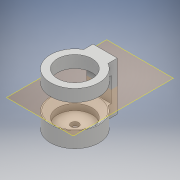
# Autodesk Inventor part: baseRotor1
Saved by Autodesk Inventor 2017 (Build 210142000, 142)
## iProperties
Created: 2017-08-06
Part Number: baseRotor1
Material: Generic
Document SubType Name: Sheet Metal
Designer: Bardo91
Density: 1 g/cm^3
Sheet Metal Rule: Default_mm
Appearance: Default
Author: Bardo91
Autodesk Inventor part; units mm, degrees
ref_plane "YZ Plane" through (0, 0, 0) normal (1, 0, 0) x (0, 1, 0)
ref_plane "XZ Plane" through (0, 0, 0) normal (0, 1, 0) x (-1, 0, 0)
ref_plane "XY Plane" through (0, 0, 0) normal (0, 0, 1) x (1, 0, 0)
sketch "Sketch1" plane through (0, 0, 0) normal (0, 0, 1) x (1, 0, 0)
  circle A0 centre (0, 0) radius 14.25
  circle A1 centre (0, 0) radius 20
  line L0 (0, 20) -> (10, 20)
  line L1 (10, 20) -> (10, 17.3205)
  line L2 (0, 20) -> (0, 20)
  line L3 (0, 20) -> (-10, 20)
  line L4 (-10, 20) -> (-10, 17.3205)
  point P0 (-20, 0)
  point P1 (20, 0)
  dimension "d0" = 28.5
  dimension "d1" = 40
  dimension "d25" = 10
  dimension "d31" = 10
  dimension "d32" = 0
  constraints: 10 end point, 5 point on circle, 2 centre point, 2 coincident, 2 perpendicular, 1 horizontal
  measures "d0" diameter of A0
  measures "d1" diameter of A1
  measures "d25" distance of L0.end L0.start
  measures "d31" distance of L0.start L3.end
  measures "d32" distance of L2.start L0.start
extrude "Extrusion1" add sketch "Sketch1" along normal blind 10
ref_plane "Work Plane1" through (0, 0, -10) normal (0, 0, 1) x (1, 0, 0)
mirror "Mirror1" about plane through (0, 0, -10) normal (0, 0, 1) of "Extrusion1"
sketch "Sketch2" plane through (0, 0, -30) normal (0, 0, -1) x (-1, 0, 0)
  circle A0 centre (0, 0) radius 14.25 projected
  circle A1 centre (0, 0) radius 20
  dimension "d11" = 40
  constraints: 1 centre point, 1 coincident
  measures "d11" diameter of A1
extrude "Extrusion2" add sketch "Sketch2" along normal blind 3 contours A0 | A1
sketch "Sketch3" plane through (0, 0, -30) normal (0, 0, 1) x (1, 0, 0)
  circle A0 centre (0, 0) radius 3.15
  dimension "d14" = 6.3
  constraints: 1 centre point, 1 coincident
  measures "d14" diameter of A0
extrude "Extrusion3" cut sketch "Sketch3" against normal blind 1
sketch "Sketch4" plane through (0, 0, -31) normal (0, 0, 1) x (1, 0, 0)
  circle A0 centre (0, 0) radius 3.15
  line L0 (0, 0) -> (0, -1.6)
  line L1 (0, -1.6) -> (-2.7134, -1.6)
  line L2 (0, -1.6) -> (2.7134, -1.6)
  dimension "d17" = 6.3
  dimension "d18" = 1.6
  constraints: 6 end point, 2 horizontal, 2 point on circle, 1 centre point, 1 coincident, 1 vertical
  measures "d17" diameter of A0
  measures "d18" distance of L0.start L0.end
extrude "Extrusion4" cut sketch "Sketch4" against normal through all contours A0 L2 L1 picked at (-0.0447, 1.5505)
sketch "Sketch6" plane through (-7.5, 20, -22) normal (0, 1, 0) x (1, 0, 0)
  line L0 (17.5, 8) -> (17.5, 8) projected
  line L1 (17.5, -22) -> (17.5, -32) projected
  line L2 (-2.5, 8) -> (17.5, 8)
  line L3 (17.5, 8) -> (17.5, -32)
  line L4 (17.5, -32) -> (-2.5, -32)
  line L5 (-2.5, -32) -> (-2.5, 8)
  point P0 (7.5, -22)
  constraints: 8 end point, 2 parallel, 1 horizontal, 1 horizontal alignment, 1 perpendicular
extrude "Extrusion6" add sketch "Sketch6" along normal blind 5
sketch "Sketch7" plane through (-7.5, 25, -22) normal (0, 1, 0) x (1, 0, 0)
  line L0 (21.75, -32) -> (-6.75, -32) projected
  line L1 (7.5, -32) -> (7.5, 8)
  line L2 (10.65, 8) -> (4.35, 8) projected
  circle A0 centre (7.5, -12) radius 4.25
  point P0 (7.5, -22)
  dimension "d28" = 8.5
  constraints: 3 midpoint, 2 end point, 1 centre point
  measures "d28" diameter of A0
extrude "Extrusion7" cut sketch "Sketch7" against normal up to next
chamfer "Chamfer1" distance 5 angle 45 1 edges at (-14.25, 0, -20)
equation "\"d4\" = d25"
equation "\"BendRadius\" = Thickness"
equation "\"BendReliefWidth\" = Thickness"
equation "\"BendReliefDepth\" = 0.5 * Thickness"
equation "\"CornerReliefSize\" = 4 * Thickness"
equation "\"MinimumRemnant\" = 2 * Thickness"
equation "\"TransitionRadius\" = BendRadius"
equation "\"JacobiRadiusSize\" = BendRadius"
equation "\"GapSize\" = Thickness"
equation "\"Thickness\" = 0.5"
body "Solid1"
